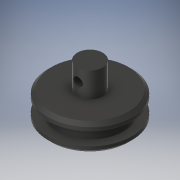
# Autodesk Inventor part: Plug
Saved by Autodesk Inventor 2017 (Build 210142000, 142)
## iProperties
Created: 2017-03-13
Part Number: Plug
Material: Acetal Resin, Black
Document SubType Name: Modeling
Designer: Joseph
Density: 1.425 g/cm^3
Appearance: Smooth - Black
Author: Joseph
Autodesk Inventor part; units mm, degrees
ref_plane "YZ Plane" through (0, 0, 0) normal (1, 0, 0) x (0, 1, 0)
ref_plane "XZ Plane" through (0, 0, 0) normal (0, 1, 0) x (-1, 0, 0)
sketch "Sketch1" plane through (0, 0, 0) normal (0, 1, 0) x (-1, 0, 0)
  circle A0 centre (0, 0) radius 15.7353
  dimension "d0" = 31.4706
  constraints: 1 centre point, 1 coincident
  measures "d0" diameter of A0
extrude "Extrusion1" add sketch "Sketch1" along normal blind 2.54
sketch "Sketch2" plane through (0, 2.54, 0) normal (0, 1, 0) x (1, 0, 0)
  circle A0 centre (0, 0) radius 12.6365
  dimension "d3" = 25.273
  constraints: 1 centre point, 1 coincident
  measures "d3" diameter of A0
extrude "Extrusion2" add sketch "Sketch2" along normal blind 4.9022
sketch "Sketch3" plane through (0, 7.4422, 0) normal (0, 1, 0) x (1, 0, 0)
  circle A0 centre (0, 0) radius 15.7353
  dimension "d6" = 31.4706
  constraints: 1 centre point, 1 coincident
  measures "d6" diameter of A0
extrude "Extrusion3" add sketch "Sketch3" along normal blind 2.54
chamfer "Chamfer1" distance 1.27 angle 45 2 edges at (-15.7353, 9.9822, 0) (15.7353, 0, 0)
sketch "Sketch4" plane through (0, 9.9822, 0) normal (0, 1, 0) x (1, 0, 0)
  circle A0 centre (0, 0) radius 4.7625
  dimension "d12" = 9.525
  constraints: 1 centre point, 1 coincident
  measures "d12" diameter of A0
extrude "Extrusion4" add sketch "Sketch4" along normal blind 9.525
ref_plane "Work Plane1" through (0, 9.9822, -4.7625) normal (0, 0, 1) x (1, 0, 0)
sketch "Sketch5" plane through (0, 9.9822, -4.7625) normal (0, 0, 1) x (1, 0, 0)
  circle A0 centre (0, 4.7625) radius 1.7526
  line L0 (-14.4653, 0) -> (14.4653, 0) projected
  point P0 (0, -9.9822)
  dimension "d15" = 3.5052
  dimension "d16" = 4.7625
  constraints: 1 centre point
  measures "d15" diameter of A0
  measures "d16" distance from line of A0.centre L0
extrude "Extrusion5" cut sketch "Sketch5" along normal blind 9.525
body "Solid1"
